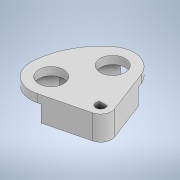
# Autodesk Inventor part: Desbalanceo
Saved by Autodesk Inventor 2022 (Build 260153000, 153)
## iProperties
Created: 2021-05-13
Part Number: Desbalanceo
Material: Generic
Document SubType Name: Modeling
Designer: juanp
Density: 1 g/cm^3
Appearance: Default
Author: juanp
Autodesk Inventor part; units mm, degrees
ref_plane "YZ Plane" through (0, 0, 0) normal (1, 0, 0) x (0, 1, 0)
ref_plane "XZ Plane" through (0, 0, 0) normal (0, 1, 0) x (-1, 0, 0)
ref_plane "XY Plane" through (0, 0, 0) normal (0, 0, 1) x (1, 0, 0)
sketch "Sketch1" plane through (0, 0, 0) normal (0, 1, 0) x (-1, 0, 0)
  arc A0 (1.2748, -0.925) -> (-1.2748, -0.925) centre (0, 0) ccw
  line L0 (1.2748, -0.925) -> (-1.2748, -0.925)
  arc A1 (-0.8639, 3.4691) -> (-3.3372, -1.2821) centre (0, 0) ccw
  line L1 (-0.8639, 3.4691) -> (21.9124, 9.141)
  line L2 (-3.3372, -1.2821) -> (5.0806, -23.1927)
  arc A2 (5.0806, -23.1927) -> (21.9124, 9.141) centre (0, 0) ccw
  circle A3 centre (16.2426, 0) radius 4.075
  circle A4 centre (9.3164, -13.3052) radius 4.075
  circle A5 centre (16.2426, 0) radius 7.5 construction
  circle A6 centre (9.3164, -13.3052) radius 7.5 construction
  line L3 (0, 0) -> (16.2426, 0) construction
  line L4 (0, 0) -> (9.3164, -13.3052) construction
  line L5 (12.4926, -6.4952) -> (8.7426, 0)
  line L6 (8.7426, 0) -> (12.4926, 6.4952)
  line L7 (12.4926, 6.4952) -> (19.9926, 6.4952)
  line L8 (19.9926, 6.4952) -> (23.7426, 0)
  line L9 (23.7426, 0) -> (19.9926, -6.4952)
  line L10 (19.9926, -6.4952) -> (12.4926, -6.4952)
  line L11 (16.8164, -13.3052) -> (13.0664, -19.8004)
  line L12 (13.0664, -19.8004) -> (5.5664, -19.8004)
  line L13 (5.5664, -19.8004) -> (1.8164, -13.3052)
  line L14 (1.8164, -13.3052) -> (5.5664, -6.81)
  line L15 (5.5664, -6.81) -> (13.0664, -6.81)
  line L16 (13.0664, -6.81) -> (16.8164, -13.3052)
  dimension "d5" = 15
  dimension "d6" = 15
  dimension "d0" = 3.15
  dimension "d1" = 2.5
  dimension "d2" = 2
  dimension "d3" = 8.15
  dimension "d4" = 8.15
  dimension "d7" = 55
  constraints: 34 end point, 7 coincident, 6 point on circle, 5 centre point, 4 horizontal, 2 tangent, 1 equal length, 1 horizontal alignment, 34 other
  measures "d0" diameter of A0
  measures "d2" radial gap between concentric circles of A0 A1
  measures "d3" diameter of A3
  measures "d4" diameter of A4
  measures "d7" angle of L3 L4
extrude "Extrusion1" add sketch "Sketch1" along normal blind 8 contours L9 L10 L5 L6 L7 L8 | L1 A2 L2 A1 | L11 L12 L13 L14 L15 L16
fillet "Fillet1" radius 8 2 edges at (-21.9124, 4, 9.141) (-5.0806, 4, -23.1927)
extrude "Extrusion2" cut sketch "Sketch1" along normal blind 5.4 contours L9 L10 L5 L6 L7 L8 | L11 L12 L13 L14 L15 L16
sketch "Sketch2" plane through (0, 0, 0) normal (0, -1, 0) x (1, 0, 0)
  arc A0 (-12.8561, -19.8004) -> (-6.2416, -19.8004) centre (-9.5488, -12.516) ccw projected
  line L0 (-6.2416, -19.8004) -> (-12.8561, -19.8004) projected
  arc A1 (-12.8561, -19.8004) -> (-6.2416, -19.8004) centre (-9.5488, -12.516) ccw projected
  line L1 (-23.6968, 0.0794) -> (-20.3388, 5.8956) projected
  arc A2 (-20.3388, 5.8956) -> (-23.6968, 0.0794) centre (-15.7295, -0.6431) ccw projected
  line L2 (-12.4926, 6.4952) -> (-8.7426, 0) projected
  line L3 (-12.4926, 6.4952) -> (-12.6949, 6.8456)
  line L4 (-13.7963, 7.1199) -> (0.8639, 3.4691) projected
  line L5 (-5.5664, -6.81) -> (-1.8164, -13.3052) projected
  line L6 (-1.8164, -13.3052) -> (-1.4955, -13.861)
  line L7 (3.3372, -1.2821) -> (-2.081, -15.385) projected
  line L8 (-1.2748, -0.925) -> (1.2748, -0.925) projected
  arc A3 (1.2748, -0.925) -> (-1.2748, -0.925) centre (0, 0) ccw projected
  line L9 (-13.1467, -19.6613) -> (-16.8164, -13.3052) projected
  line L10 (-16.8164, -13.3052) -> (-13.0664, -6.81) projected
  line L11 (-13.0664, -6.81) -> (-5.5664, -6.81) projected
  line L12 (-5.5664, -6.81) -> (-1.8164, -13.3052) projected
  line L13 (-1.8164, -13.3052) -> (-5.2596, -19.2689) projected
  arc A4 (-5.2596, -19.2689) -> (-2.081, -15.385) centre (-9.5488, -12.516) ccw projected
  line L14 (3.3372, -1.2821) -> (-2.081, -15.385) projected
  arc A5 (3.3372, -1.2821) -> (0.8639, 3.4691) centre (0, 0) ccw projected
  line L15 (-13.7963, 7.1199) -> (0.8639, 3.4691) projected
  arc A6 (-13.7963, 7.1199) -> (-19.3413, 6.4952) centre (-15.7295, -0.6431) ccw projected
  line L16 (-19.3413, 6.4952) -> (-12.4926, 6.4952) projected
  line L17 (-12.4926, 6.4952) -> (-8.7426, 0) projected
  line L18 (-8.7426, 0) -> (-12.4926, -6.4952) projected
  line L19 (-12.4926, -6.4952) -> (-19.9926, -6.4952) projected
  line L20 (-19.9926, -6.4952) -> (-23.7082, -0.0597) projected
  arc A7 (-23.7082, -0.0597) -> (-23.7228, -0.9698) centre (-15.7295, -0.6431) ccw projected
  arc A8 (-23.7228, -0.9698) -> (-14.4013, -18.8763) centre (0, 0) ccw projected
  arc A9 (-14.4013, -18.8763) -> (-13.1467, -19.6613) centre (-9.5488, -12.516) ccw projected
  point P0 (-2.081, -15.385)
  point P1 (-13.7963, 7.1199)
  constraints: 4 end point, 2 collinear, 2 point on line
extrude "Extrusion3" cut sketch "Sketch2" against normal up to surface (5.4 mm away) contours L0 A0 | A2 L1 | L16 A6 L4 L3 | L7 A4 L13 L6 | A3 L8
body "Solid1"
